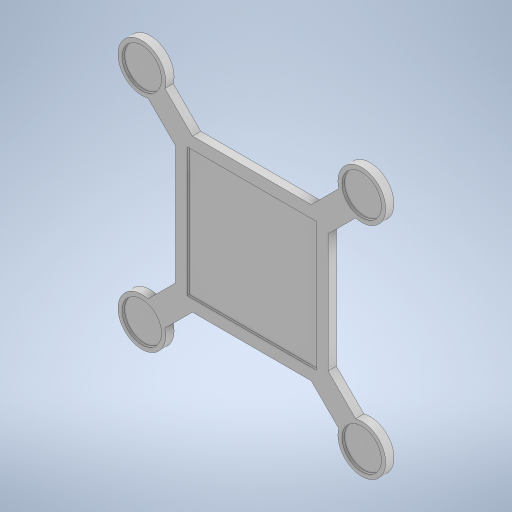
# Autodesk Inventor part: holder
Saved by Autodesk Inventor 2024 (Build 280153000, 153)
## iProperties
Created: 2023-08-08
Part Number: holder
Material: Generic
Document SubType Name: Modeling
Designer: Pintu
Density: 1 g/cm^3
Appearance: Default
Author: Pintu
Autodesk Inventor part; units mm, degrees
ref_plane "YZ Plane" through (0, 0, 0) normal (1, 0, 0) x (0, 1, 0)
ref_plane "XZ Plane" through (0, 0, 0) normal (0, 1, 0) x (-1, 0, 0)
ref_plane "XY Plane" through (0, 0, 0) normal (0, 0, 1) x (1, 0, 0)
sketch "Sketch1" plane through (0, 0, 0) normal (0, 0, 1) x (1, 0, 0)
  line L0 (-32, 32) -> (32, 32)
  line L1 (32, 32) -> (32, -32)
  line L2 (32, -32) -> (-32, -32)
  line L3 (-32, -32) -> (-32, 32)
  line L4 (-32, 32) -> (32, -32) construction
  line L5 (32, 32) -> (-32, -32) construction
  point P0 (0, 0)
  dimension "d0" = 64
  dimension "d1" = 64
  constraints: 12 end point, 2 midpoint, 2 parallel, 1 horizontal, 1 perpendicular
  measures "d0" distance of L1.end L2.end
  measures "d1" distance of L0.end L1.end
extrude "Extrusion1" add sketch "Sketch1" along normal blind 3.5
sketch "Sketch2" plane through (0, 0, 3.5) normal (0, 0, 1) x (1, 0, 0)
  line L0 (-27, 27) -> (27, 27)
  line L1 (27, 27) -> (27, -27)
  line L2 (27, -27) -> (-27, -27)
  line L3 (-27, -27) -> (-27, 27)
  line L4 (-27, 27) -> (27, -27) construction
  line L5 (27, 27) -> (-27, -27) construction
  point P0 (0, 0)
  dimension "d4" = 54
  dimension "d5" = 54
  constraints: 12 end point, 2 midpoint, 2 parallel, 1 horizontal, 1 perpendicular
  measures "d4" distance of L1.end L2.end
  measures "d5" distance of L0.end L1.end
extrude "Extrusion2" cut sketch "Sketch2" against normal blind 0.7
sketch "Sketch3" plane through (0, 0, 0) normal (0, 0, 1) x (1, 0, 0)
  line L0 (-32, 32) -> (-32, -32) projected
  line L1 (32, -32) -> (32, 32) projected
  line L2 (-32, -32) -> (32, -32) projected
  line L3 (32, -32) -> (32, 32) projected
  line L4 (32, 32) -> (-32, 32) projected
  line L5 (-32, 32) -> (-46.1421, 46.1421)
  circle A0 centre (-46.1421, 46.1421) radius 10
  line L6 (-36.4829, 43.5539) -> (-24.9289, 32)
  line L7 (32, 32) -> (-32, 32) projected
  line L8 (-43.5539, 36.4829) -> (-32, 24.9289)
  line L9 (32, 32) -> (46.1421, 46.1421)
  circle A1 centre (46.1421, 46.1421) radius 10
  line L10 (43.5539, 36.4829) -> (32, 24.9289)
  line L11 (36.4829, 43.5539) -> (24.9289, 32)
  line L12 (-32, -32) -> (-46.1421, -46.1421)
  circle A2 centre (-46.1421, -46.1421) radius 10
  line L13 (-36.4829, -43.5539) -> (-23.7494, -30.8205)
  line L14 (-43.5539, -36.4829) -> (-32, -24.9289)
  line L15 (32, -32) -> (46.1421, -46.1421)
  circle A3 centre (46.1421, -46.1421) radius 10
  line L16 (43.5539, -36.4829) -> (32, -24.9289)
  line L17 (36.4829, -43.5539) -> (24.9289, -32)
  point P0 (0, 0)
  point P1 (-30.7059, 37.777)
  point P2 (-24.9289, -32)
  dimension "d28" = 135
  dimension "d29" = 20
  dimension "d30" = 20
  dimension "d31" = 5
  dimension "d32" = 5
  dimension "d33" = 135
  dimension "d34" = 20
  dimension "d35" = 20
  dimension "d36" = 5
  dimension "d37" = 5
  dimension "d38" = 20
  dimension "d39" = 135
  dimension "d40" = 20
  dimension "d41" = 5
  dimension "d42" = 5
  dimension "d43" = 20
  dimension "d44" = 135
  dimension "d45" = 20
  dimension "d46" = 5
  dimension "d47" = 5
  constraints: 24 end point, 8 parallel, 8 point on circle, 7 point on line, 4 centre point, 4 coincident, 1 midpoint
  measures "d28" angle of L0 L5
  measures "d29" distance of L0.start L5.end
  measures "d30" diameter of A0
  measures "d31" distance from line of point (-30.706, 37.777) L5
  measures "d32" distance between parallel lines of L5 L8
  measures "d33" angle of L1 L9
  measures "d34" distance of L1.end L9.end
  measures "d35" diameter of A1
  measures "d36" distance between parallel lines of L11 L9
  measures "d37" distance between parallel lines of L10 L9
  measures "d38" distance of L0.end L12.end
  measures "d39" angle of L2 L12
  measures "d40" diameter of A2
  measures "d41" distance between parallel lines of L12 L14
  measures "d42" distance between parallel lines of L13 L12
  measures "d43" distance of L1.start L15.end
  measures "d44" angle of L3 L15
  measures "d45" diameter of A3
  measures "d46" distance between parallel lines of L16 L15
  measures "d47" distance between parallel lines of L15 L17
extrude "Extrusion3" add sketch "Sketch3" along normal blind 3.5 contours L5 A0 L6 L4 | L0 L8 A0 L5 | A0 | L0 L12 A2 L14 | L11 A1 L9 L4 | L2 L13 A2 L12 | A2 | L9 A1 L10 L1 | A1 | L2 L15 A3 L17 | L16 A3 L15 L1 | A3
sketch "Sketch4" plane through (0, 0, 3.5) normal (0, 0, 1) x (1, 0, 0)
  arc A0 (-36.4829, 43.5539) -> (-43.5539, 36.4829) centre (-46.1421, 46.1421) ccw projected
  arc A1 (43.5539, 36.4829) -> (36.4829, 43.5539) centre (46.1421, 46.1421) ccw projected
  arc A2 (36.4829, -43.5539) -> (43.5539, -36.4829) centre (46.1421, -46.1421) ccw projected
  arc A3 (-43.5539, -36.4829) -> (-36.4829, -43.5539) centre (-46.1421, -46.1421) ccw projected
  circle A4 centre (-46.1421, 46.1421) radius 8.25
  circle A5 centre (46.1421, 46.1421) radius 8.25
  circle A6 centre (46.1421, -46.1421) radius 8.25
  circle A7 centre (-46.1421, -46.1421) radius 8.25
  point P0 (0, 0)
  dimension "d50" = 16.5
  dimension "d51" = 16.5
  dimension "d52" = 16.5
  dimension "d53" = 16.5
  constraints: 4 centre point, 4 coincident
  measures "d50" diameter of A4
  measures "d51" diameter of A5
  measures "d52" diameter of A6
  measures "d53" diameter of A7
extrude "Extrusion4" cut sketch "Sketch4" against normal blind 1
body "Solid1"
